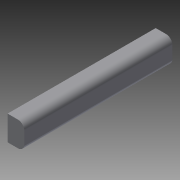
# Autodesk Inventor part: Robot Bumper (31 inches)
Saved by Autodesk Inventor 2014 (Build 180170000, 170)
## iProperties
Created: 2016-01-25
Part Number: Robot Bumper (31 inches)
Material: Generic
Document SubType Name: Modeling
Designer: shawnsargent
Density: 1 g/cm^3
Appearance: Default
Author: shawnsargent
Autodesk Inventor part; units mm, degrees
ref_plane "YZ Plane" through (0, 0, 0) normal (1, 0, 0) x (0, 1, 0)
ref_plane "XZ Plane" through (0, 0, 0) normal (0, 1, 0) x (-1, 0, 0)
ref_plane "XY Plane" through (0, 0, 0) normal (0, 0, 1) x (1, 0, 0)
sketch "Sketch1" plane through (0, 0, 0) normal (0, 0, 1) x (1, 0, 0)
  line L0 (0, 0) -> (0, 132.08)
  line L1 (0, 132.08) -> (25.4, 132.08)
  line L2 (0, 66.04) -> (63.5, 66.04)
  line L3 (0, 132.08) -> (0, 66.04)
  line L4 (0, 99.06) -> (31.75, 99.06)
  arc A0 (63.5, 99.06) -> (55.043838, 120.634513) centre (31.75, 99.06) ccw
  line L5 (0, 66.04) -> (0, 0)
  arc A1 (54.194148, 10.562869) -> (63.5, 33.02) centre (31.75, 33.02) ccw
  line L6 (63.5, 28.211314) -> (63.5, 99.06)
  arc A2 (59.079555, 115.220381) -> (25.4, 132.08) centre (28.846947, 96.896052) ccw
  line L7 (0, 0) -> (25.4, 0)
  arc A3 (25.4, 0) -> (63.5, 28.211314) centre (28.813006, 35.223762) ccw
  line L8 (0, 132.08) -> (-25.4, 132.08)
  line L9 (0, 1.27) -> (0, 132.08)
  line L10 (0, 132.08) -> (-25.4, 132.08)
  line L11 (-25.4, 132.08) -> (-25.4, 1.27)
  line L12 (-25.4, 0) -> (0, 0)
  line L13 (0, 0) -> (0, 132.08)
  line L14 (0, 132.08) -> (-25.4, 132.08)
  line L15 (-25.4, 132.08) -> (-25.4, 0)
  dimension "d0" = 132.08
  dimension "d1" = 25.4
  dimension "d2" = 63.5
  dimension "d3" = 25.4
  dimension "d4" = 25.4
  constraints: 32 end point, 11 point on circle, 7 parallel, 4 centre point, 4 perpendicular, 3 tangent, 2 midpoint, 2 point on line, 1 coincident, 1 collinear, 1 horizontal, 1 vertical
  measures "d0" distance of L0.start L0.end
  measures "d1" distance of L0.end L1.end
  measures "d2" distance of L2.start L2.end
  measures "d3" distance of L0.start L7.end
  measures "d4" distance of L0.end L8.end
sketch "Sketch1 outline for Extrusion1" plane through (0, 0, 0) normal (0, 0, 1) x (1, 0, 0)
  line L0 (-25.4, 0) -> (25.4, 0)
  arc A0 (25.4, 0) -> (63.5, 28.211314) centre (28.813006, 35.223762) ccw
  line L1 (63.5, 28.211314) -> (63.5, 99.06)
  arc A1 (63.5, 99.06) -> (59.079555, 115.220381) centre (31.75, 99.06) ccw
  arc A2 (59.079555, 115.220381) -> (25.4, 132.08) centre (28.846947, 96.896052) ccw
  line L2 (25.4, 132.08) -> (-25.4, 132.08)
  line L3 (-25.4, 132.08) -> (-25.4, 0)
extrude "Extrusion1" add sketch "Sketch1 outline for Extrusion1" along normal blind 787.4
body "Solid1"
